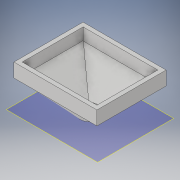
# Autodesk Inventor part: Container Final
Saved by Autodesk Inventor 2019 (Build 230136000, 136)
## iProperties
Created: 2019-10-20
Part Number: Container Final
Material: Generic
Document SubType Name: Modeling
Designer: sudhanva
Density: 1 g/cm^3
Appearance: Default
Author: sudhanva
Autodesk Inventor part; units mm, degrees
ref_plane "YZ Plane" through (0, 0, 0) normal (1, 0, 0) x (0, 1, 0)
ref_plane "XZ Plane" through (0, 0, 0) normal (0, 1, 0) x (-1, 0, 0)
ref_plane "XY Plane" through (0, 0, 0) normal (0, 0, 1) x (1, 0, 0)
sketch "Sketch1" plane through (0, 0, 0) normal (0, 0, 1) x (1, 0, 0)
  line L0 (-150, 75) -> (150, 75)
  line L1 (150, 75) -> (150, 25)
  line L2 (150, 25) -> (-150, 25)
  line L3 (-150, 25) -> (-150, 75)
  point P0 (0, 0)
  dimension "d0" = 300
  dimension "d1" = 75
  dimension "d2" = 50
  dimension "d3" = 150
  constraints: 8 end point, 2 parallel, 1 horizontal, 1 perpendicular
  measures "d0" distance of L0.end L0.start
  measures "d1" distance from line of point (0, 0) L0
  measures "d2" distance of L1.end L0.end
  measures "d3" distance from line of point (0, 0) L1
extrude "Extrusion1" add sketch "Sketch1" along normal blind 250
ref_plane "Work Plane1" through (-150, -75, 0) normal (0, -1, 0) x (1, 0, 0)
sketch "Sketch2" plane through (-150, -75, 0) normal (0, -1, 0) x (1, 0, 0)
  circle A0 centre (150, 125) radius 35
  line L0 (0, 0) -> (0, 250) projected
  point P0 (150, 0)
  dimension "d7" = 70
  dimension "d8" = 125
  dimension "d9" = 150
  constraints: 1 centre point
  measures "d7" diameter of A0
  measures "d8" distance of point (150, 0) A0.centre
  measures "d9" distance from line of L0 A0.centre
loft "Loft1" add profiles "Sketch2" section 1 edges at (0, 25, 0) (150, 25, 125) (0, 25, 250) (-150, 25, 125)
shell "Shell1" thickness 15 removed faces 1 at (-50, 75, 83.3333)
sketch "Sketch3" plane through (0.0006, -60, 101.0339) normal (0, 1, 0) x (0.7163363, 0, 0.6977552)
  point P0 (-70.4973, 72.3738)
  point P1 (16.1192, -16.5493)
hole "Hole1" at (0, -60, 124.136) direction (0, -1, 0) diameter 70 depth 9 tip angle 118
body "Solid1"
